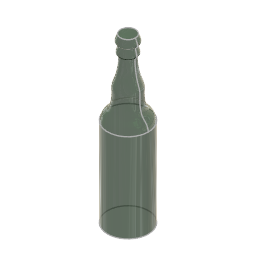
Day 2 - Glass Soda Bottle (Autodesk Fusion 360 design; units mm, degrees)
part number: 2025-06-14-20-15-48-329
part number: 2025-06-14-20-19-33-888
Autodesk Fusion 360 part; units mm, degrees
sketch "Sketch1" plane through (0, 0, 0) normal (0, 1, 0) x (1, 0, 0) in component "Bottle"
  line L0 (0, 0) -> (0, -240)
  line L1 (0, 0) -> (30, 0)
  line L2 (30, 0) -> (30, -130)
  spline S0 degree 5 poles (30, -130) (29.8911, -130.5608) (29.6614, -131.6461) (29.2815, -133.1654) (28.7044, -134.9739) (27.8669, -136.8804) (26.9195, -138.459) (25.8744, -139.7638) (24.7526, -140.8843) (23.5862, -141.9599) (22.4163, -143.1602) (21.2884, -144.6484) (20.2477, -146.551) (19.3351, -148.9237) (18.583, -151.7224) (18.0129, -154.8339) (17.633, -158.1027) (17.4359, -161.3581) (17.3962, -164.4417) (17.4673, -167.2356) (17.5805, -169.6872) (17.6391, -171.8435) (17.534, -173.8397) (17.171, -175.8649) (16.4935, -178.1356) (15.5084, -180.865) (14.3074, -184.2371) (13.1037, -188.3759) (12.0293, -193.1332) (11.1733, -198.2075) (10.58, -203.1971) (10.2606, -207.6787) (10.2004, -211.2758) (10.3669, -213.7285) (10.7184, -214.9719) (11.2096, -215.1886) (11.8066, -214.9306) (12.4604, -214.9774) (12.9754, -215.7375) (13.1054, -217.2446) (12.7516, -219.3187) (12.0686, -221.6661) (11.3364, -223.9539) (10.8657, -225.8842) (10.8942, -227.2659) (11.4773, -228.0952) (12.4073, -228.6102) (13.3581, -229.1543) (14.0293, -230.0378) (14.2332, -231.4554) (13.8541, -233.5263) (13.0405, -235.7514) (12.135, -237.7482) (11.4002, -239.2251) (11, -240) knots 0 0 0 0 0 0 0.02 0.04 0.06 0.08 0.1 0.12 0.14 0.16 0.18 0.2 0.22 0.24 0.26 0.28 0.3 0.32 0.34 0.36 0.38 0.4 0.42 0.44 0.46 0.48 0.5 0.52 0.54 0.56 0.58 0.6 0.62 0.64 0.66 0.68 0.7 0.72 0.74 0.76 0.78 0.8 0.82 0.84 0.86 0.88 0.9 0.92 0.94 0.96 0.98 1 1 1 1 1 1
  line L3 (18.9255, -170.8772) -> (11, -194)
  line L4 (0, -240) -> (11, -240)
  point P0 (25.508, -140.0984)
  point P1 (20.3633, -146.4867)
  point P2 (17.5073, -168)
  point P3 (14.9627, -182.4386)
  point P4 (11, -215)
  point P5 (12, -215)
  point P6 (13, -217)
  point P7 (11, -227)
  point P8 (13, -229)
  dimension "d1" = 240
  dimension "d2" = 30
  dimension "d3" = 130
  dimension "d7" = 11
  constraint coincident L0.start L1.start
  constraint vertical L0
  constraint perpendicular L0 L1
  constraint perpendicular L1 L2
  constraint midpoint P3 L3
  measures "d1" distance of L0.start L0.end
  measures "d2" distance of L0.start L1.end
  measures "d3" distance of L1.end L2.end
  measures "d7" distance of L0.end S0.end
revolve "Revolve1" add sketch "Sketch1" angle 360 about axis through (0, 0, 0) along (0, 0, 1) in component "Bottle"
fillet "Fillet1" [suppressed] in component "Bottle"
shell "Shell1" [suppressed] in component "Bottle"
fillet "Fillet2" [suppressed] in component "Bottle"
component "Bottle" placed x (1, 0, 0) y (0, 1, 0) z (0, 0, 1) at (0, 0, 0)
